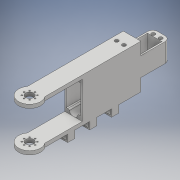
# Autodesk Inventor part: Brazo_p1_new
Saved by Autodesk Inventor 2018 (Build 220112000, 112)
## iProperties
Created: 2017-11-07
Part Number: Brazo_p1_new
Material: Generic
Document SubType Name: Modeling
Designer: Bardo91
Density: 1 g/cm^3
Appearance: Default
Author: Bardo91
Autodesk Inventor part; units mm, degrees
ref_plane "YZ Plane" through (0, 0, 0) normal (1, 0, 0) x (0, 1, 0)
ref_plane "XZ Plane" through (0, 0, 0) normal (0, 1, 0) x (-1, 0, 0)
ref_plane "XY Plane" through (0, 0, 0) normal (0, 0, 1) x (1, 0, 0)
sketch "Sketch1" plane through (0, 0, 0) normal (0, 0, 1) x (1, 0, 0)
  line L0 (0, 0) -> (24, 0)
  line L1 (24, 0) -> (24, 190)
  line L2 (24, 190) -> (0, 190)
  line L3 (0, 190) -> (0, 0)
  dimension "d0" = 24
  dimension "d1" = 190
  constraints: 8 end point, 1 horizontal, 1 parallel, 1 perpendicular, 1 vertical
  measures "d0" distance of L0.start L0.end
  measures "d1" distance of L0.end L1.end
extrude "base" add sketch "Sketch1" along normal blind 60
sketch "Sketch2" plane through (24, 0, 0) normal (1, 0, 0) x (0, 0, -1)
  line L0 (0, 0) -> (-5, 0)
  line L1 (0, 0) -> (-60, 0) projected
  line L2 (-5, 0) -> (-5, 70)
  line L3 (-5, 70) -> (-55, 70)
  line L4 (-55, 70) -> (-55, 0)
  line L5 (-55, 0) -> (-5, 0)
  dimension "d4" = 5
  dimension "d5" = 70
  dimension "d6" = 50
  constraints: 10 end point, 2 perpendicular, 2 point on line, 1 horizontal, 1 vertical
  measures "d4" distance of L0.start L0.end
  measures "d5" distance of L0.end L2.end
  measures "d6" distance of L2.end L3.end
extrude "shape_base" cut sketch "Sketch2" against normal up to next
sketch "Sketch3" plane through (24, 70, 5) normal (0, -1, 0) x (1, 0, 0)
  line L0 (0, 50) -> (0, 0) projected
  line L1 (0, 25) -> (0, 44.5)
  line L2 (0, 44.5) -> (-24, 44.5)
  line L3 (-24, 44.5) -> (-24, 5.5)
  line L4 (-24, 0) -> (-24, 50) projected
  line L5 (-24, 5.5) -> (0, 5.5)
  line L6 (-12, 44.5) -> (-2, 44.5)
  line L7 (-2, 44.5) -> (-2, 5.5)
  line L8 (-12, 44.5) -> (-22, 44.5)
  line L9 (-22, 44.5) -> (-22, 5.5)
  circle A0 centre (-12, 44.5) radius 6
  circle A1 centre (-12, 5.5) radius 6
  point P0 (-24, -5)
  dimension "d9" = 19.5
  dimension "d10" = 39
  dimension "d11" = 10
  dimension "d12" = 10
  dimension "d13" = 12
  dimension "d14" = 12
  constraints: 16 end point, 7 point on line, 4 perpendicular, 3 midpoint, 2 centre point, 1 coincident
  measures "d9" distance of L1.start L1.end
  measures "d10" distance of L2.end L3.end
  measures "d11" distance of L6.start L6.end
  measures "d12" distance of L6.start L8.end
  measures "d13" diameter of A0
  measures "d14" diameter of A1
extrude "internal_servo_slot" cut sketch "Sketch3" against normal blind 111 contours L7 L5 A1 L9 L2 A0 | A0 L2 | L2 A0 | A1 L5 | L5 A1
sketch "Sketch4" plane through (24, 0, 0) normal (1, 0, 0) x (0, 0, -1)
  line L0 (-60, 0) -> (-60, 190) projected
  line L1 (-60, 190) -> (-60, 150)
  line L2 (0, 190) -> (0, 150)
  line L3 (0, 0) -> (0, 190) projected
  line L4 (-60, 150) -> (-43, 150)
  line L5 (-43, 150) -> (-43, 190)
  line L6 (0, 190) -> (-60, 190) projected
  line L7 (-60, 190) -> (-43, 190)
  line L8 (0, 190) -> (-17, 190)
  line L9 (-17, 190) -> (-17, 150)
  line L10 (-17, 150) -> (0, 150)
  dimension "d17" = 40
  dimension "d18" = 40
  dimension "d19" = 17
  dimension "d20" = 17
  dimension "d21" = 40
  constraints: 16 end point, 5 point on line, 1 collinear, 1 horizontal, 1 perpendicular
  measures "d17" distance of L0.end L1.end
  measures "d18" distance of L2.start L2.end
  measures "d19" distance of L1.end L4.end
  measures "d20" distance of L2.start L8.end
  measures "d21" distance of L8.end L9.end
extrude "shape_end" cut sketch "Sketch4" against normal up to next
sketch "Sketch5" plane through (24, 150, 17) normal (0, 0, -1) x (-1, 0, 0)
  line L0 (0, 40) -> (24, 40) projected
  line L1 (0, 40) -> (0, 34)
  line L2 (0, 0) -> (0, 40) projected
  line L3 (0, 34) -> (7, 34)
  circle A0 centre (7, 34) radius 2.5
  line L4 (24, 40) -> (24, 34)
  line L5 (24, 34) -> (17, 34)
  circle A1 centre (17, 34) radius 2.5
  line L6 (7, 34) -> (17, 34)
  point P0 (24, -150)
  dimension "d24" = 6
  dimension "d25" = 7
  dimension "d26" = 5
  dimension "d27" = 6
  dimension "d28" = 7
  dimension "d29" = 5
  constraints: 10 end point, 2 centre point, 2 coincident, 1 horizontal, 1 perpendicular, 1 point on line, 1 vertical
  measures "d24" distance of L0.start L1.end
  measures "d25" distance of L1.end L3.end
  measures "d26" diameter of A0
  measures "d27" distance of L0.end L4.end
  measures "d28" distance of L4.end L5.end
  measures "d29" diameter of A1
extrude "servo_attach_end" cut sketch "Sketch5" against normal up to next contours A0 L6 L3 | L3 L6 A0 | A1 L6 L5 | L5 L6 A1
sketch "Sketch6" plane through (0, 0, 0) normal (0, 0, -1) x (-1, 0, 0)
  line L0 (0, 0) -> (-24, 0) projected
  line L1 (-12, 0) -> (-12, 10)
  circle A0 centre (-12, 10) radius 5.5
  line L2 (-12, 10) -> (-12, 17.5)
  circle A1 centre (-12, 17.5) radius 1
  circle A2 centre (-17.3033, 15.3033) radius 1
  circle A3 centre (-19.5, 10) radius 1
  circle A4 centre (-17.3033, 4.6967) radius 1
  circle A5 centre (-12, 2.5) radius 1
  circle A6 centre (-6.6967, 4.6967) radius 1
  circle A7 centre (-4.5, 10) radius 1
  circle A8 centre (-6.6967, 15.3033) radius 1
  dimension "d32" = 10
  dimension "d33" = 11
  dimension "d34" = 7.5
  dimension "d35" = 2
  dimension "d38" = 360
  constraints: 9 centre point, 4 end point, 2 coincident, 2 vertical, 1 midpoint, 17 other
  measures "d32" distance of L1.start L1.end
  measures "d33" diameter of A0
  measures "d34" distance of L2.start L2.end
  measures "d35" diameter of A1
extrude "servo_attach_base" cut sketch "Sketch6" against normal through all
fillet "Fillet1" radius 7 6 edges at (24, 0, 57.5) (0, 0, 57.5) (24, 0, 2.5) (0, 0, 2.5) (24, 190, 30) (0, 190, 30)
sketch "Sketch7" plane through (0, 0, 0) normal (0, 0, -1) x (-1, 0, 0)
  circle A0 centre (-7, 184) radius 2.5 projected
  line L0 (-7, 184) -> (-7, 133.9)
  line L1 (-7, 133.9) -> (-17, 133.9)
  line L2 (-6, 70) -> (-6, 150) projected
  line L3 (-7, 133.9) -> (3, 133.9) construction
  circle A1 centre (-17, 133.9) radius 2.5
  circle A2 centre (-7, 133.9) radius 2.5
  point P0 (0, 0)
  dimension "d43" = 50.1
  dimension "d44" = 10
  dimension "d45" = 180
  dimension "d46" = 5
  dimension "d47" = 5
  constraints: 4 end point, 2 centre point, 2 coincident, 2 horizontal, 1 collinear, 4 other
  measures "d43" distance of A0.centre L1.start
  measures "d44" distance of L1.start L1.end
  measures "d45" angle of L1 L3
  measures "d46" diameter of A1
  measures "d47" diameter of A2
extrude "Extrusion7" cut sketch "Sketch7" against normal through all contours A2 L2 L1 L0 | L0 L1 A2 | A2 L2 | A1
sketch "Sketch8" plane through (0, 0, 0) normal (0, 0, -1) x (-1, 0, 0)
  line L0 (0, 150) -> (-24, 150) projected
  line L1 (-24, 150) -> (-24, 120)
  line L2 (-24, 7) -> (-24, 150) projected
  line L3 (-24, 120) -> (-24, 110)
  line L4 (-24, 110) -> (-24, 90)
  line L5 (-24, 90) -> (-24, 80)
  line L6 (-24, 80) -> (-24, 60)
  line L7 (-24, 60) -> (-24, 50)
  line L8 (-24, 70) -> (-24, 7) projected
  line L9 (-24, 50) -> (0, 50)
  line L10 (0, 50) -> (0, 60)
  line L11 (0, 60) -> (-24, 60)
  line L12 (-24, 80) -> (0, 80)
  line L13 (0, 80) -> (0, 90)
  line L14 (0, 90) -> (-24, 90)
  line L15 (-24, 110) -> (0, 110)
  line L16 (0, 110) -> (0, 120)
  line L17 (0, 120) -> (-24, 120)
  point P0 (0, 0)
  dimension "d50" = 30
  dimension "d51" = 10
  dimension "d52" = 20
  dimension "d53" = 10
  dimension "d54" = 20
  dimension "d55" = 10
  constraints: 30 end point, 10 point on line, 5 perpendicular, 2 parallel
  measures "d50" distance of L0.end L1.end
  measures "d51" distance of L1.end L3.end
  measures "d52" distance of L3.end L4.end
  measures "d53" distance of L4.end L5.end
  measures "d54" distance of L5.end L6.end
  measures "d55" distance of L6.end L7.end
extrude "Extrusion8" add sketch "Sketch8" along normal blind 10
sketch "Sketch9" plane through (0, 120, 0) normal (0, 1, 0) x (1, 0, 0)
  line L0 (0, 0) -> (0, 10) projected
  line L1 (0, 0) -> (2, 0)
  line L2 (0, 0) -> (24, 0) projected
  line L3 (2, 0) -> (2, 8)
  line L4 (2, 8) -> (22, 8)
  line L5 (22, 8) -> (22, 0)
  line L6 (22, 0) -> (2, 0)
  dimension "d58" = 2
  dimension "d59" = 8
  dimension "d60" = 20
  constraints: 10 end point, 3 perpendicular, 2 point on line, 1 horizontal
  measures "d58" distance of L0.start L1.end
  measures "d59" distance of L1.end L3.end
  measures "d60" distance of L3.end L4.end
extrude "Extrusion9" cut sketch "Sketch9" against normal up to surface (70 mm away)
sketch "Sketch10" plane through (0, 0, 60) normal (0, 0, 1) x (1, 0, 0)
  circle A0 centre (12, 10) radius 5.5 projected
  circle A1 centre (12, 10) radius 15
  point P0 (0, 0)
  dimension "d63" = 30
  constraints: 1 centre point, 1 coincident
  measures "d63" diameter of A1
extrude "Extrusion10" add sketch "Sketch10" against normal up to surface (5 mm away)
sketch "Sketch11" plane through (0, 0, 0) normal (0, 0, -1) x (-1, 0, 0)
  circle A0 centre (-12, 10) radius 5.5 projected
  circle A1 centre (-12, 10) radius 15
  point P0 (0, 0)
  dimension "d66" = 30
  constraints: 1 centre point, 1 coincident
  measures "d66" diameter of A1
extrude "Extrusion11" add sketch "Sketch11" against normal up to surface (5 mm away)
extrude "Extrusion12" cut sketch "Sketch6" against normal through all contours A5 L1 | L1 A5 | A1 | A2 | A3 | A4 | A6 | A7 | A8
fillet "Fillet2" radius 2 8 edges at (18, 100.8044, 10.5) (18, 143.0956, 10.5) (6, 100.8044, 10.5) (6, 143.0956, 10.5) (18, 100.8044, 49.5) (18, 143.0956, 49.5) (6, 100.8044, 49.5) (6, 143.0956, 49.5)
body "Solid1"
